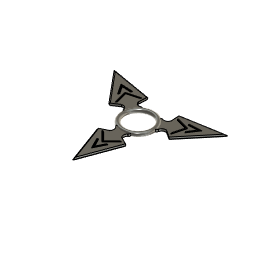
Throwing star v2 (Autodesk Fusion 360 design; units mm, degrees)
Autodesk Fusion 360 part; units mm, degrees
sketch "Sketch2" plane through (0, 0, 0) normal (0, 0, 1) x (1, 0, 0) in component "sTAR"
  line L0 (-6, -5) -> (-3, -5)
  line L1 (-3, -8) -> (-7, -10)
  line L2 (-7, -10) -> (0, -29)
  line L3 (0, -29) -> (7, -10)
  line L4 (7, -10) -> (3, -8)
  line L5 (3, -5) -> (6, -5)
  line L6 (6, -5) -> (-6, -5)
  line L7 (-3, -8) -> (0, -8) construction
  line L8 (0, -8) -> (3, -8) construction
  line L9 (-7, -10) -> (7, -10) construction
  arc A0 (3, -5) -> (3, -8) centre (4.4, -6.5) ccw
  arc A1 (-3, -8) -> (-3, -5) centre (-4.2571, -6.5) ccw
  arc A2 (2.3482, -6.5) -> (-2.2929, -6.5) centre (0.0241, -11152046.7524) ccw construction
  constraint horizontal L0
  constraint parallel L8 L9
  constraint midpoint A0 A2.start
extrude "Extrude1" add sketch "Sketch2" along normal blind 1 makes body 1 in component "sTAR"
chamfer "Chamfer1" distance 0.5 angle 45 2 edges at (-3.5, -19.5, 1) (-3.5, -19.5, 0) on bodies 1 in component "sTAR"
chamfer "Chamfer2" distance 0.5 angle 45 2 edges at (3.6332, -19.1384, 1) (3.6332, -19.1384, 0) on bodies 1 in component "sTAR"
move_body "Move1" bodies 1 to x (1, 0, 0) y (0, 1, 0) z (0, 0, 1) at (0, -17, 0) in component "sTAR"
sketch "Sketch3" plane through (0, 0, 0) normal (1, 0, 0) x (0, 1, 0) in component "sTAR"
  circle A0 centre (7, 0) radius 1
  dimension "d7" = 2
  measures "d7" diameter of A0
revolve "Revolve2" add sketch "Sketch3" angle 360 about axis through (0, 0, 1.75) along (0, 0, 1) separate body makes body 2 in component "sTAR"
move_body "Move2" bodies 1 to x (1, 0, 0) y (0, 1, 0) z (0, 0, 1) at (0, 14, 0) in component "sTAR"
move_body "Move3" bodies 1 to x (1, 0, 0) y (0, 1, 0) z (0, 0, 1) at (0, 0, -0.5) in component "sTAR"
sketch "Sketch5" plane through (0, 0, 0) normal (0, 0, 1) x (1, 0, 0) in component "sTAR"
  arc A0 (-3.5, -7.1) -> (-3, -8) centre (-2.0651, -6.8917) ccw
  arc A1 (3, -8) -> (3.4899, -7.094) centre (2.5961, -7.1961) ccw
  line L0 (3.4899, -7.094) -> (-3.5, -7.1)
  line L1 (3, -8) -> (-3, -8)
  dimension "d9" = 1.03
  constraint horizontal L1
  measures "d9" distance of A1.start A1.end
extrude "Extrude2" add sketch "Sketch5" along normal blind 0.5 bodies 2 1 in component "sTAR"
extrude "Extrude3" add sketch "Sketch5" against normal blind 0.5 bodies 2 in component "sTAR"
delete_face "DeleteFace1" 1 faces at (-2.9202, -7.1064, -0.7304) on bodies 2 in component "sTAR"
sketch "Sketch1" plane through (0, 0, 0) normal (1, 0, 0) x (0, 1, 0) in component "Ring"
  circle A0 centre (-7.1, 0) radius 1
  dimension "d16" = 2
  measures "d16" diameter of A0
revolve "Revolve1" add sketch "Sketch1" angle 360 about axis through (0, 0, 1.75) along (0, 0, 1) separate body makes body 3 in component "Ring"
sketch "Sketch6" plane through (0, 0, 0.5) normal (0, 0, 1) x (-1, 0, 0) in component "sTAR"
  arc A0 (3, 11) -> (3, 8) centre (4.2571, 9.5) ccw
  line L0 (3, 11) -> (6.55, 12.775)
  line L1 (6.55, 12.775) -> (0, 30.5537)
  line L2 (0, 30.5537) -> (-6.55, 12.775)
  line L3 (-6.55, 12.775) -> (-3, 11)
  arc A1 (-3, 8) -> (-3, 11) centre (-4.4, 9.5) ccw
  arc A2 (-3, 8) -> (-3.4899, 7.094) centre (-2.5961, 7.1961) ccw
  line L4 (-3.4899, 7.094) -> (3.5, 7.1)
  arc A3 (3.5, 7.1) -> (3, 8) centre (2.0651, 6.8917) ccw
  line L5 (2.5, 17.5) -> (0, 22.5)
  line L6 (0, 22.5) -> (-2.5, 17.5)
  line L7 (-2.5, 17.5) -> (-2, 17.5)
  line L8 (-2, 17.5) -> (0, 21.5)
  line L9 (0, 21.5) -> (2, 17.5)
  line L10 (2, 17.5) -> (2.5, 17.5)
  line L11 (4.5, 13) -> (0, 17.5)
  line L12 (0, 17.5) -> (-4.5, 13)
  line L13 (-4.5, 13) -> (-4, 13)
  line L14 (-4, 13) -> (0, 17)
  line L15 (0, 17) -> (4, 13)
  line L16 (4, 13) -> (4.5, 13)
  constraint horizontal L7
  constraint parallel L6 L8
  constraint parallel L5 L9
  constraint parallel L7 L10
  constraint perpendicular L11 L12
  constraint parallel L10 L13
  constraint perpendicular L11 L14
  constraint perpendicular L14 L15
  constraint parallel L13 L16
extrude "Extrude4" cut sketch "Sketch6" against normal blind 0.25 contours L5 L6 L7 L8 L9 L10 bodies 2 in component "sTAR"
extrude "Extrude5" cut sketch "Sketch6" against normal blind 0.25 contours L11 L12 L13 L14 L15 L16 bodies 2 in component "sTAR"
chamfer "Chamfer3" distance 0.125 angle 45 6 edges at (1.25, -20, 0.5) (2.25, -17.5, 0.5) (1, -19.5, 0.5) (-1, -19.5, 0.5) (-2.25, -17.5, 0.5) (-1.25, -20, 0.5) on bodies 2 in component "sTAR"
chamfer "Chamfer4" distance 0.125 angle 45 6 edges at (-1, -19.5, 0.25) (-2.25, -17.5, 0.25) (-1.25, -20, 0.25) (1.25, -20, 0.25) (2.25, -17.5, 0.25) (1, -19.5, 0.25) on bodies 2 in component "sTAR"
chamfer "Chamfer5" distance 0.125 angle 45 6 edges at (2, -15, 0.5) (2.25, -15.25, 0.5) (-2, -15, 0.5) (-2.25, -15.25, 0.5) (-4.25, -13, 0.5) (4.25, -13, 0.5) on bodies 2 in component "sTAR"
chamfer "Chamfer6" distance 0.125 angle 45 6 edges at (2, -15, 0.25) (-2, -15, 0.25) (-4.25, -13, 0.25) (-2.25, -15.25, 0.25) (2.25, -15.25, 0.25) (4.25, -13, 0.25) on bodies 2 in component "sTAR"
sketch "Sketch7" plane through (0, 0, -0.5) normal (0, 0, -1) x (1, 0, 0) in component "sTAR"
  arc A0 (-3, 8) -> (-3.5, 7.1) centre (-2.0651, 6.8917) ccw
  line L0 (-3.5, 7.1) -> (3.4899, 7.094)
  arc A1 (3.4899, 7.094) -> (3, 8) centre (2.5961, 7.1961) ccw
  arc A2 (3, 11) -> (3, 8) centre (4.4, 9.5) ccw
  line L1 (3, 11) -> (6.55, 12.775)
  line L2 (6.55, 12.775) -> (0, 30.5537)
  line L3 (0, 30.5537) -> (-6.55, 12.775)
  line L4 (-6.55, 12.775) -> (-3, 11)
  arc A3 (-3, 8) -> (-3, 11) centre (-4.2571, 9.5) ccw
  line L5 (0, 22.5) -> (2.5, 17.5)
  line L6 (2.5, 17.5) -> (2, 17.5)
  line L7 (2, 17.5) -> (0, 21.5)
  line L8 (0, 21.5) -> (-2, 17.5)
  line L9 (-2, 17.5) -> (-2.5, 17.5)
  line L10 (-2.5, 17.5) -> (0, 22.5)
  line L11 (0, 17.5) -> (4.5, 13)
  line L12 (4.5, 13) -> (4, 13)
  line L13 (4, 13) -> (0, 17)
  line L14 (0, 17) -> (-4, 13)
  line L15 (-4, 13) -> (-4.5, 13)
  line L16 (-4.5, 13) -> (0, 17.5)
  constraint horizontal L6
  constraint parallel L5 L7
  constraint parallel L6 L9
  constraint parallel L8 L10
  constraint parallel L9 L12
  constraint parallel L11 L13
  constraint perpendicular L13 L14
  constraint parallel L12 L15
  constraint perpendicular L11 L16
extrude "Extrude6" cut sketch "Sketch7" against normal blind 0.25 contours L5 L6 L7 L8 L9 L10 bodies 2 in component "sTAR"
extrude "Extrude7" cut sketch "Sketch7" against normal blind 0.25 contours L11 L12 L13 L14 L15 L16 bodies 2 in component "sTAR"
chamfer "Chamfer7" distance 0.125 angle 45 23 edges at (-1, -19.5, -0.25) (-1, -19.5, -0.5) (-2.25, -17.5, -0.5) (-2.25, -17.5, -0.25) (-1.25, -20, -0.5) (-1.25, -20, -0.25) (1.25, -20, -0.5) (1.25, -20, -0.25) (1, -19.5, -0.5) (1, -19.5, -0.25) (2.25, -17.5, -0.5) (2.25, -17.5, -0.25) (-2, -15, -0.5) (-2.25, -15.25, -0.25) (-2, -15, -0.25) (2, -15, -0.5) (2, -15, -0.25) (2.25, -15.25, -0.5) (2.25, -15.25, -0.25) (4.25, -13, -0.25) (4.25, -13, -0.5) (-4.25, -13, -0.25) (-4.25, -13, -0.5) on bodies 2 in component "sTAR"
component_pattern "component pattern"
component "sTAR" placed x (1, 0, 0) y (0, 1, 0) z (0, 0, 1) at (0, 0, 0)
component "Ring" placed x (1, 0, 0) y (0, 1, 0) z (0, 0, 1) at (0, 0, 0)
component "sTAR" placed x (-0.5, 0.866025, 0) y (-0.866025, -0.5, 0) z (0, 0, 1) at (0, 0, 0)
component "sTAR" placed x (-0.5, -0.866025, 0) y (0.866025, -0.5, 0) z (0, 0, 1) at (0, 0, 0)
